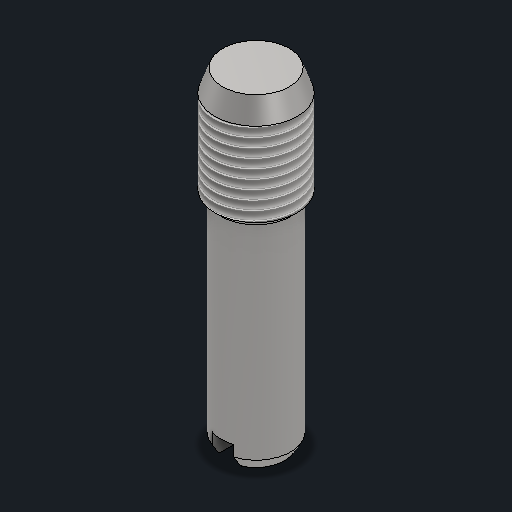
# Autodesk Inventor part: 0.16 Shaft
Saved by Autodesk Inventor 2025.1 (Build 291241020, 241B)
## iProperties
Created: 2025-05-15
Part Number: 0.16 Shaft
Material: Stainless Steel
Document SubType Name: Modeling
Designer: Joshua Eah
Density: 8 g/cm^3
Appearance: Semi-Polished
Author: Joshua Eah
Autodesk Inventor part; units mm, degrees
ref_plane "YZ Plane" through (0, 0, 0) normal (1, 0, 0) x (0, 1, 0)
ref_plane "XZ Plane" through (0, 0, 0) normal (0, 1, 0) x (-1, 0, 0)
ref_plane "XY Plane" through (0, 0, 0) normal (0, 0, 1) x (1, 0, 0)
sketch "Sketch1" plane through (0, 0, 0) normal (0, 1, 0) x (-1, 0, 0)
  circle A0 centre (0, 0) radius 2.032
  line L0 (-0.635, 2.032) -> (0.635, 2.032)
  line L1 (0.635, 2.032) -> (0.635, -2.032)
  line L2 (0.635, -2.032) -> (-0.635, -2.032)
  line L3 (-0.635, -2.032) -> (-0.635, 2.032)
  line L4 (-0.635, 2.032) -> (0.635, -2.032) construction
  line L5 (0.635, 2.032) -> (-0.635, -2.032) construction
  dimension "d0" = 4.064
  dimension "d10" = 1.27
  constraints: 12 end point, 2 midpoint, 2 parallel, 1 centre point, 1 coincident, 1 horizontal, 1 perpendicular, 1 tangent
  measures "d0" diameter of A0
  measures "d10" distance of L1.end L2.end
extrude "Extrusion1" add sketch "Sketch1" along normal blind 12.954 contours A0 L1 | L1 A0 L3 | L3 A0
sketch "Sketch2" plane through (0, 12.954, 0) normal (0, 1, 0) x (1, 0, 0)
  circle A0 centre (0, 0) radius 2.413
  dimension "d5" = 4.826
  constraints: 1 centre point, 1 coincident
  measures "d5" diameter of A0
extrude "Extrusion2" add sketch "Sketch2" along normal blind 6.1595
thread "Thread2" size "10-48 UNS" class "2A" standard "ANSI Unified Screw Threads" length 19.1262
chamfer "Chamfer1" distance 0.381 angle 45 1 edges at (2.032, 12.954, 0)
chamfer "Chamfer2" distance 1.27 angle 20 1 edges at (-2.413, 19.1135, 0) measured on face at (2.4052, 17.0603, 0.1942)
chamfer "Chamfer3" distance 0.635 angle 30 1 edges at (2.032, 0, 0) measured on face at (-2.0254, 8.3823, -0.1635)
extrude "Extrusion3" cut sketch "Sketch1" along normal blind 1.27 contours L1 A0 L3 | A0 L0 L1 | L1 L2 A0 | A0 L3 L0 | L2 L3 A0
body "Solid1"
